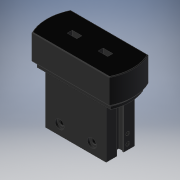
# Autodesk Inventor part: 539636 HGP-16-A-B-SSK---(0_1_ZYL)
Saved by Autodesk Inventor 2019 (Build 230136000, 136)
## iProperties
Created: 2023-03-06
Part Number: 539636 HGP-16-A-B-SSK---(0_1_ZYL)
Material: Generic
Catalog Web Link: www.cadenas.de
Description: HGP-(ZYL)-parallel gripper
Vendor: FESTO
Document SubType Name: Modeling
Designer: psAdmin
Manufacturer: FESTO
Mass: 80.8406 g
Surface Area: 154.928 cm^2
Volume: 80.8406 cm^3
Density: 1 g/cm^3
Appearance: PSOLRGB-175-175-175
Category: PARTsolutions
Company: FESTO
Title: 539636 HGP-16-A-B-SSK
Author: Cadenas PARTsolutions
Comments: parallel gripper
PSOL_IDENT_0: {$CADENAS_DATA/23d-libs/festo/parts/h/hgp/parts/hgp_zyl.prj},216 {VTYP=3D},{NB=539636 HGP-16-A-B-SSK
PSOL_IDENT_1: ---(0_1_ZYL)},{LINA=539636 HGP-16-A-B-SSK},{NN=HGP-(ZYL)},{DATE=10.09.2021 08:18:21},{GEOMDATE=11.03
PSOL_IDENT_2: .2020 13:19:07},{VERSION=},{LINEID=210},{WBVAR=HUBST,ZBH},{WBNUMERIC=HUBST,ZBH}  {NB=539636 HGP-16-A
PSOL_IDENT_3: -B-SSK---(0_1_ZYL)},{LINA=539636 HGP-16-A-B-SSK},{KT=3},{TNR=539636},{TYP=HGP-16-A-B-SSK},{KDM=116},
PSOL_IDENT_4: {HUBST=0},{ZBH=1},{B1=47.000},{B2=25.000},{B3=16.400},{B4=43.800},{B5=46.400},{B6=10.000},{B8=67.000
PSOL_IDENT_5: },{D2=M 4},{D3=7.000},{D4=M 4},{D5=3.300},{D6=3.000},{EE=M 3},{H1=83.000},{H2=20.500},{H3=21.900},{H
PSOL_IDENT_6: 4=7.500},{H5=7.000},{H6=4.000},{H7=11.000},{H8=5.500},{H9=10.000},{H11=38.100},{L1=22.000},{L2=5.700
PSOL_IDENT_7: },{L3=10.000},{L6=0.000},{L6S=30.000},{T1=1.600},{T2=7.000},{T3=7.500},{T4=3.500},{T5=1.400},{T6=4.5
PSOL_IDENT_8: 00},{EEP=3.000},{KDREE=2.459},{D2P=4.000},{KDR2=3.242},{D4P=4.000},{KDR5=3.242},{LHUB=5.000},{VERS=3
PSOL_IDENT_9: .000},{ZT=-ZH},{V=0}
NB: 539636 HGP-16-A-B-SSK---(0_1_ZYL)
NN: HGP-(ZYL)
NT: parallel gripper
NBSYN: $TNR. $TYP.---($HUBST._$ZBH._ZYL)
LINA: 539636 HGP-16-A-B-SSK
CATALOG: Festo
TNR: 539636
TYP: HGP-16-A-B-SSK
KDM: 116
HUBST: 0
ZBH: With centring sleeves (2xZBH)
B1: 47
B2: 25
B3: 16.4
B4: 43.8
B5: 46.4
B6: 10
B8: 67
D2: M 4
D3: 7
D4: M 4
D5: 3.3
D6: 3
EE: M 3
H1: 83
H2: 20.5
H3: 21.9
H4: 7.5
H5: 7
H6: 4
H7: 11
H8: 5.5
H9: 10
H11: 38.1
L1: 22
L2: 5.7
L3: 10
L6: 0
L6S: 30
T1: 1.6
T2: 7
T3: 7.5
T4: 3.5
T5: 1.4
T6: 4.5
EEP: 3
KDREE: 2.459
D2P: 4
KDR2: 3.242
D4P: 4
KDR5: 3.242
V: 0
SUPPLIER: FESTO
ARTICLENO: 539636 HGP-16-A-B-SSK---(0_1_ZYL)
BOMINFO: 539636 HGP-16-A-B-SSK
CREATOR: CADENAS GmbH
Autodesk Inventor part; units mm, degrees
ref_plane "YZ Plane" through (0, 0, 0) normal (1, 0, 0) x (0, 1, 0)
ref_plane "XZ Plane" through (0, 0, 0) normal (0, 1, 0) x (-1, 0, 0)
ref_plane "XY Plane" through (0, 0, 0) normal (0, 0, 1) x (1, 0, 0)
sketch "Sketch_1" plane through (0, 0, 0) normal (0, 0, 1) x (1, 0, 0)
  line L0 (-23.5, 0) -> (23.5, 0)
  line L1 (23.5, 0) -> (23.5, 62.5)
  line L2 (23.5, 62.5) -> (-23.5, 62.5)
  line L3 (-23.5, 62.5) -> (-23.5, 0)
  constraints: 8 end point
extrude "Extrusion1" add sketch "Sketch_1" along normal mid plane 22
sketch "Sketch2" plane through (23.5, 0, 11) normal (1, 0, 0) x (0, 0, -1)
  point P0 (16.7, 4)
hole "Hole1" at (23.5, 4, -5.7) direction (-1, 0, 0) diameter 2.459 depth 3.5 countersink diameter 3 countersink angle 90 thread size "M3x0.5" class "6H" standard "ISO Metric profile"
sketch "Sketch3" plane through (23.5, 0, 11) normal (1, 0, 0) x (0, 0, -1)
  point P0 (16.7, 11)
hole "Hole2" at (23.5, 11, -5.7) direction (-1, 0, 0) diameter 2.459 depth 3.5 countersink diameter 3 countersink angle 90 thread size "M3x0.5" class "6H" standard "ISO Metric profile"
sketch "Sketch_7" plane through (0, 0, 0) normal (0, 0, 1) x (1, 0, 0)
  line L0 (12.5, 0) -> (12.5, 8.6)
  line L1 (12.5, 8.6) -> (14.121, 8.6)
  line L2 (14.121, 8.6) -> (14.121, 1.979)
  line L3 (14.121, 1.979) -> (14.5, 1.6)
  line L4 (14.5, 1.6) -> (16, 1.6)
  line L5 (16, 1.6) -> (16, 0)
  line L6 (16, 0) -> (12.5, 0)
  line L7 (12.5, 0) -> (12.5, 8.6)
  constraints: 16 end point
revolve "Revolution1" cut sketch "Sketch_7" angle 360 about axis through (12.5, 0, 0) along (0, 1, 0)
thread "Thread1" size "M4x0.7" class "6H" standard "ISO Metric profile" full length
sketch "Sketch_8" plane through (0, 0, 0) normal (0, 1, 0) x (-1, 0, 0)
  line L0 (-19.1, -2.85) -> (-19.1, 2.85)
  arc A0 (-19.1, 2.85) -> (-19.5, 3.25) centre (-19.5, 2.85) ccw
  line L1 (-19.5, 3.25) -> (-22.1, 3.25)
  arc A1 (-22.1, 3.25) -> (-22.3, 3.05) centre (-22.1, 3.05) ccw
  line L2 (-22.3, 3.05) -> (-22.3, 2.8)
  arc A2 (-22.5, 2.6) -> (-22.3, 2.8) centre (-22.5, 2.8) ccw
  line L3 (-22.5, 2.6) -> (-23.2, 2.6)
  arc A3 (-23.6, 3) -> (-23.2, 2.6) centre (-23.2, 3) ccw
  line L4 (-23.6, 3) -> (-23.6, -3)
  arc A4 (-23.2, -2.6) -> (-23.6, -3) centre (-23.2, -3) ccw
  line L5 (-23.2, -2.6) -> (-22.5, -2.6)
  arc A5 (-22.3, -2.8) -> (-22.5, -2.6) centre (-22.5, -2.8) ccw
  line L6 (-22.3, -2.8) -> (-22.3, -3.05)
  arc A6 (-22.3, -3.05) -> (-22.1, -3.25) centre (-22.1, -3.05) ccw
  line L7 (-22.1, -3.25) -> (-19.5, -3.25)
  arc A7 (-19.5, -3.25) -> (-19.1, -2.85) centre (-19.5, -2.85) ccw
  constraints: 16 end point, 16 point on circle, 8 centre point
extrude "Extrusion2" cut sketch "Sketch_8" along normal mid plane 81.2
sketch "Sketch_9" plane through (0, 0, 0) normal (0, 1, 0) x (-1, 0, 0)
  line L0 (23.6, -3) -> (23.6, 3)
  arc A0 (23.2, 2.6) -> (23.6, 3) centre (23.2, 3) ccw
  line L1 (23.2, 2.6) -> (22.5, 2.6)
  arc A1 (22.3, 2.8) -> (22.5, 2.6) centre (22.5, 2.8) ccw
  line L2 (22.3, 2.8) -> (22.3, 3.05)
  arc A2 (22.3, 3.05) -> (22.1, 3.25) centre (22.1, 3.05) ccw
  line L3 (22.1, 3.25) -> (19.5, 3.25)
  arc A3 (19.5, 3.25) -> (19.1, 2.85) centre (19.5, 2.85) ccw
  line L4 (19.1, 2.85) -> (19.1, -2.85)
  arc A4 (19.1, -2.85) -> (19.5, -3.25) centre (19.5, -2.85) ccw
  line L5 (19.5, -3.25) -> (22.1, -3.25)
  arc A5 (22.1, -3.25) -> (22.3, -3.05) centre (22.1, -3.05) ccw
  line L6 (22.3, -3.05) -> (22.3, -2.8)
  arc A6 (22.5, -2.6) -> (22.3, -2.8) centre (22.5, -2.8) ccw
  line L7 (22.5, -2.6) -> (23.2, -2.6)
  arc A7 (23.6, -3) -> (23.2, -2.6) centre (23.2, -3) ccw
  constraints: 16 end point, 16 point on circle, 8 centre point
extrude "Extrusion3" cut sketch "Sketch_9" along normal mid plane 81.2
sketch "Sketch_4" plane through (12.5, 0, 0) normal (1, 0, 0) x (0, 0, -1)
  line L0 (0, 7.5) -> (-11, 7.5)
  line L1 (-11, 7.5) -> (-11, 11)
  line L2 (-11, 11) -> (-9.4, 11)
  line L3 (-9.4, 11) -> (-9.4, 9.5)
  line L4 (-9.4, 9.5) -> (-9.021, 9.121)
  line L5 (-9.021, 9.121) -> (0, 9.121)
  line L6 (0, 9.121) -> (0, 7.5)
  line L7 (0, 7.5) -> (-11, 7.5)
  constraints: 16 end point
revolve "Revolution2" cut sketch "Sketch_4" angle 360 about axis through (12.5, 7.5, 0) along (0, 0, 1)
thread "Thread2" size "M4x0.7" class "6H" standard "ISO Metric profile" length 5.521
sketch "Sketch_14" plane through (12.5, 0, 0) normal (1, 0, 0) x (0, 0, -1)
  line L0 (11, 7.5) -> (0, 7.5)
  line L1 (0, 7.5) -> (0, 9.121)
  line L2 (0, 9.121) -> (9.021, 9.121)
  line L3 (9.021, 9.121) -> (9.4, 9.5)
  line L4 (9.4, 9.5) -> (9.4, 11)
  line L5 (9.4, 11) -> (11, 11)
  line L6 (11, 11) -> (11, 7.5)
  line L7 (11, 7.5) -> (0, 7.5)
  constraints: 16 end point
revolve "Revolution3" cut sketch "Sketch_14" angle 360 about axis through (12.5, 7.5, -11) along (0, 0, 1)
sketch "Sketch_5" plane through (-12.5, 0, 0) normal (1, 0, 0) x (0, 0, -1)
  line L0 (0, 7.5) -> (-11, 7.5)
  line L1 (-11, 7.5) -> (-11, 11)
  line L2 (-11, 11) -> (-9.4, 11)
  line L3 (-9.4, 11) -> (-9.4, 9.5)
  line L4 (-9.4, 9.5) -> (-9.021, 9.121)
  line L5 (-9.021, 9.121) -> (0, 9.121)
  line L6 (0, 9.121) -> (0, 7.5)
  line L7 (0, 7.5) -> (-11, 7.5)
  constraints: 16 end point
revolve "Revolution4" cut sketch "Sketch_5" angle 360 about axis through (-12.5, 7.5, 0) along (0, 0, 1)
thread "Thread3" size "M4x0.7" class "6H" standard "ISO Metric profile" length 5.521
sketch "Sketch_15" plane through (-12.5, 0, 0) normal (1, 0, 0) x (0, 0, -1)
  line L0 (11, 7.5) -> (0, 7.5)
  line L1 (0, 7.5) -> (0, 9.121)
  line L2 (0, 9.121) -> (9.021, 9.121)
  line L3 (9.021, 9.121) -> (9.4, 9.5)
  line L4 (9.4, 9.5) -> (9.4, 11)
  line L5 (9.4, 11) -> (11, 11)
  line L6 (11, 11) -> (11, 7.5)
  line L7 (11, 7.5) -> (0, 7.5)
  constraints: 16 end point
revolve "Revolution5" cut sketch "Sketch_15" angle 360 about axis through (-12.5, 7.5, -11) along (0, 0, 1)
thread "Thread4" size "M4x0.7" class "6H" standard "ISO Metric profile" length 5.521
sketch "Sketch_6" plane through (0, 0, 0) normal (0, 0, 1) x (1, 0, 0)
  line L0 (-12.5, 8.6) -> (-12.5, 0)
  line L1 (-12.5, 0) -> (-16, 0)
  line L2 (-16, 0) -> (-16, 1.6)
  line L3 (-16, 1.6) -> (-14.5, 1.6)
  line L4 (-14.5, 1.6) -> (-14.121, 1.979)
  line L5 (-14.121, 1.979) -> (-14.121, 8.6)
  line L6 (-14.121, 8.6) -> (-12.5, 8.6)
  line L7 (-12.5, 8.6) -> (-12.5, 0)
  constraints: 16 end point
revolve "Revolution6" cut sketch "Sketch_6" angle 360 about axis through (-12.5, 8.6, 0) along (0, -1, 0)
thread "Thread5" size "M4x0.7" class "6H" standard "ISO Metric profile" length 6.621
sketch "Skizze_3" plane through (0, 0, 0) normal (1, 0, 0) x (0, 1, 0)
  arc A0 (43.3071, 15) -> (42.9536, 14.8536) centre (43.3071, 14.5) ccw
  line L0 (42.9536, 14.8536) -> (40.6, 12.5)
  line L1 (40.6, 12.5) -> (38.6, 12.5)
  arc A1 (38.6, 12.5) -> (38.1, 12) centre (38.6, 12) ccw
  line L2 (38.1, 12) -> (38.1, -12)
  arc A2 (38.1, -12) -> (38.6, -12.5) centre (38.6, -12) ccw
  line L3 (38.6, -12.5) -> (40.6, -12.5)
  line L4 (40.6, -12.5) -> (42.9536, -14.8536)
  arc A3 (42.9536, -14.8536) -> (43.3071, -15) centre (43.3071, -14.5) ccw
  line L5 (43.3071, -15) -> (62, -15)
  arc A4 (62, -15) -> (62.5, -14.5) centre (62, -14.5) ccw
  line L6 (62.5, -14.5) -> (62.5, 14.5)
  arc A5 (62.5, 14.5) -> (62, 15) centre (62, 14.5) ccw
  line L7 (62, 15) -> (43.3071, 15)
  constraints: 16 end point, 12 point on circle, 6 centre point
extrude "Extrusion4" add sketch "Skizze_3" along normal mid plane 67
sketch "Skizze_4" plane through (0, 0, 0) normal (0, 0, 1) x (1, 0, 0)
  line L0 (0, 38.1) -> (0, 62.5)
  line L1 (30.5, 38.1) -> (50.25, 38.1)
  line L2 (50.25, 38.1) -> (50.25, 62.5)
  line L3 (50.25, 62.5) -> (33, 62.5)
  arc A0 (33.5, 62) -> (33, 62.5) centre (33, 62) ccw
  line L4 (33.5, 62) -> (33.5, 43.3071)
  arc A1 (33.3536, 42.9536) -> (33.5, 43.3071) centre (33, 43.3071) ccw
  line L5 (33.3536, 42.9536) -> (31, 40.6)
  line L6 (31, 40.6) -> (31, 38.6)
  arc A2 (30.5, 38.1) -> (31, 38.6) centre (30.5, 38.6) ccw
  constraints: 14 end point, 6 point on circle, 3 centre point
revolve "Revolution7" cut sketch "Skizze_4" angle 90 mid plane about axis through (0, 38.1, 0) along (0, 1, 0)
sketch "Skizze_5" plane through (0, 0, 0) normal (0, 0, 1) x (1, 0, 0)
  line L0 (0, 62.5) -> (0, 38.1)
  line L1 (-50.25, 62.5) -> (-50.25, 38.1)
  line L2 (-50.25, 38.1) -> (-30.5, 38.1)
  arc A0 (-31, 38.6) -> (-30.5, 38.1) centre (-30.5, 38.6) ccw
  line L3 (-31, 38.6) -> (-31, 40.6)
  line L4 (-31, 40.6) -> (-33.3536, 42.9536)
  arc A1 (-33.5, 43.3071) -> (-33.3536, 42.9536) centre (-33, 43.3071) ccw
  line L5 (-33.5, 43.3071) -> (-33.5, 62)
  arc A2 (-33, 62.5) -> (-33.5, 62) centre (-33, 62) ccw
  line L6 (-33, 62.5) -> (-50.25, 62.5)
  constraints: 14 end point, 6 point on circle, 3 centre point
revolve "Revolution8" cut sketch "Skizze_5" angle 90 mid plane about axis through (0, 62.5, 0) along (0, -1, 0)
sketch "Sketch_10" plane through (-8.2, 0, 0) normal (1, 0, 0) x (0, 0, -1)
  arc A0 (-2, 58.5) -> (2, 58.5) centre (0, 53.9174) ccw
  line L0 (2, 58.5) -> (2, 62.5)
  line L1 (2, 62.5) -> (-2, 62.5)
  line L2 (-2, 62.5) -> (-2, 58.5)
  constraints: 6 end point, 2 point on circle, 1 centre point
extrude "Extrusion5" cut sketch "Sketch_10" against normal blind 7.5
sketch "Sketch_11" plane through (8.2, 0, 0) normal (1, 0, 0) x (0, 0, -1)
  arc A0 (-2, 58.5) -> (2, 58.5) centre (0, 53.9174) ccw
  line L0 (2, 58.5) -> (2, 62.5)
  line L1 (2, 62.5) -> (-2, 62.5)
  line L2 (-2, 62.5) -> (-2, 58.5)
  constraints: 6 end point, 2 point on circle, 1 centre point
extrude "Extrusion6" cut sketch "Sketch_11" along normal blind 7.5
ref_plane "JAW_1_XY" through (-8.2, 62.5, 0) normal (-1, 0, 0) x (0, 0, 1)
ref_plane "JAW_1_YZ" through (-8.2, 62.5, 0) normal (0, 0, 1) x (0, 1, 0)
ref_plane "JAW_1_ZX" through (-8.2, 62.5, 0) normal (0, 1, 0) x (-1, 0, 0)
ref_plane "JAW_2_XY" through (8.2, 62.5, 0) normal (1, 0, 0) x (0, 0, -1)
ref_plane "JAW_2_YZ" through (8.2, 62.5, 0) normal (0, 0, -1) x (0, 1, 0)
ref_plane "JAW_2_ZX" through (8.2, 62.5, 0) normal (0, 1, 0) x (1, 0, 0)
ref_plane "ZBH_1_XY" through (-12.5, 1.6, 0) normal (0, -1, 0) x (-1, 0, 0)
ref_plane "ZBH_1_YZ" through (-12.5, 1.6, 0) normal (-1, 0, 0) x (0, 0, -1)
ref_plane "ZBH_1_ZX" through (-12.5, 1.6, 0) normal (0, 0, -1) x (0, -1, 0)
ref_plane "ZBH_2_XY" through (12.5, 1.6, 0) normal (0, -1, 0) x (-1, 0, 0)
ref_plane "ZBH_2_YZ" through (12.5, 1.6, 0) normal (-1, 0, 0) x (0, 0, -1)
ref_plane "ZBH_2_ZX" through (12.5, 1.6, 0) normal (0, 0, -1) x (0, -1, 0)
body "Solid1"
